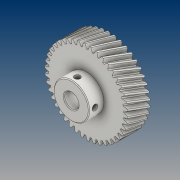
# Autodesk Inventor part: Final_Rang_Lon
Saved by Autodesk Inventor 2021 (Build 250183000, 183)
## iProperties
CustomPartVersion: 1
Created: 2024-04-07
Part Number: Final_Rang_Lon
Material: Steel
Document SubType Name: Modeling
Designer: Admin
Categories: <?xml version="1.0" encoding="UTF-16"?> <MemberInstance><Categories><FamilyTemplate><FamilyTemplateParameter ValueType="xs:double" Id="1" ObjectReferenceKey="da_z" ObjectType="kUserParameterObject"/><FamilyTemplateParameter ValueType="xs:double" Id="2" ObjectReferenceKey="da_b" ObjectType="kUserParameterObject"/><FamilyTemplateParameter ValueType="xs:double" Id="3" ObjectReferenceKey="da_beta" ObjectType="kUserParameterObject"/><FamilyTemplateParameter ValueType="xs:double" Id="4" ObjectReferenceKey="da_da" ObjectType="kUserParameterObject"/><FamilyTemplateParameter ValueType="xs:double" Id="5" ObjectReferenceKey="da_aw" ObjectType="kUserParameterObject"/><FamilyTemplateParameter ValueType="xs:string" Id="6" ObjectReferenceKey="EAIAABAAAACIAQAAAAAAAIAAAAAAAAAA" ObjectType="83910656" SubObjectId="SurfaceGeometry"/></FamilyTemplate><ParamToTemplateMap><ParamToTemplate CategoryParameter="//CategoryParameter[@InternalName='046C89C9-8512-4d59-83FE-43B91F4F132A']" TemplateParameter="1"/><ParamToTemplate CategoryParameter="//CategoryParameter[@InternalName='2552DF32-E462-4b46-AEBF-C6C7768E72AC']" TemplateParameter="2"/><ParamToTemplate CategoryParameter="//CategoryParameter[@InternalName='C9EE641D-15FC-4fae-A226-E94C4372FDD7']" TemplateParameter="3"/><ParamToTemplate><ParamToTemplate CategoryParameter="//CategoryParameter[@InternalName='00B6519A-459B-49c7-AD84-2E56D39A5744']" ConstantValue="-1.106123"/></ParamToTemplate><ParamToTemplate><ParamToTemplate CategoryParameter="//CategoryParameter[@InternalName='04B31F0E-C7A6-4894-AA32-9629BEFACF47']" ConstantValue="1.000000"/></ParamToTemplate><ParamToTemplate><ParamToTemplate CategoryParameter="//CategoryParameter[@InternalName='43CBEC2E-7847-49e7-A936-2F7889FCB2D9']" ConstantValue="0.250000"/></ParamToTemplate><ParamToTemplate><ParamToTemplate CategoryParameter="//CategoryParameter[@InternalName='B1EFC894-105D-4ebd-86BF-FA20ED196853']" ConstantValue="0.350000"/></ParamToTemplate><ParamToTemplate><ParamToTemplate CategoryParameter="//CategoryParameter[@InternalName='51175063-3D10-4879-93E8-6246FE8B403D']" ConstantValue="2060000000.000000"/></ParamToTemplate><ParamToTemplate><ParamToTemplate CategoryParameter="//CategoryParameter[@InternalName='A3A52E27-4454-46a9-B0BD-C932399B70AF']" ConstantValue="0.300000"/></ParamToTemplate><ParamToTemplate><ParamToTemplate CategoryParameter="//CategoryParameter[@InternalName='91B76062-C214-41d9-B1B9-14D2AB99603D']" ConstantValue="0.125000"/></ParamToTemplate><ParamToTemplate><ParamToTemplate CategoryParameter="//CategoryParameter[@InternalName='374E806E-8B8A-4dda-A9AA-1039D6500AD2']" ConstantValue="8.000000"/></ParamToTemplate><ParamToTemplate><ParamToTemplate CategoryParameter="//CategoryParameter[@InternalName='2D373A89-B862-43d6-8D0B-0CBF12AB9F6C']" ConstantValue="0.366519"/></ParamToTemplate><ParamToTemplate CategoryParameter="//CategoryParameter[@InternalName='37777632-D6A2-4fac-9D53-DB8ACD95C989']" TemplateParameter="4"/><ParamToTemplate CategoryParameter="//CategoryParameter[@InternalName='FD1017F1-B727-4f7e-9707-0F86F1FF9423']" TemplateParameter="5"/><ParamToTemplate><ParamToTemplate CategoryParameter="//CategoryParameter[@InternalName='9E1B4470-B2D3-4ff1-B813-535BB4CDF51A']" ConstantValue="3520000.000000"/></ParamToTemplate><ParamToTemplate><ParamToTemplate CategoryParameter="//CategoryParameter[@InternalName='F8452263-BFF6-458c-9FB1-07C4B99E95CD']" ConstantValue="11400000.000000"/></ParamToTemplate><ParamToTemplate><ParamToTemplate CategoryParameter="//CategoryParameter[@InternalName='3E3BB259-FD49-497f-8171-6EBC954A3479']" ConstantValue="2.000000"/></ParamToTemplate><ParamToTemplate CategoryParameter="//CategoryParameter[@InternalName='27C3BAF2-7550-4e4b-AE2C-0DB134B7D9B7']" TemplateParameter="6"/></ParamToTemplateMap><Category DisplayName="Gear" InternalName="DC85795E-93AB-48d5-8EEE-5A27447B64BD" Mnemonic="Gear"><CategoryParameter DisplayName="z" InternalName="046C89C9-8512-4d59-83FE-43B91F4F132A" Mnemonic="z"/><CategoryParameter DisplayName="b" InternalName="2552DF32-E462-4b46-AEBF-C6C7768E72AC" Mnemonic="b"/><CategoryParameter DisplayName="||b|" InternalName="C9EE641D-15FC-4fae-A226-E94C4372FDD7" Mnemonic="beta"/><CategoryParameter DisplayName="x" InternalName="00B6519A-459B-49c7-AD84-2E56D39A5744" Mnemonic="x"/><CategoryParameter DisplayName="a*" InternalName="04B31F0E-C7A6-4894-AA32-9629BEFACF47" Mnemonic="a"/><CategoryParameter DisplayName="c*" InternalName="43CBEC2E-7847-49e7-A936-2F7889FCB2D9" Mnemonic="c"/><CategoryParameter DisplayName="r|.f|*" InternalName="B1EFC894-105D-4ebd-86BF-FA20ED196853" Mnemonic="rf"/><CategoryParameter DisplayName="E" InternalName="51175063-3D10-4879-93E8-6246FE8B403D" Mnemonic="E"/><CategoryParameter DisplayName="||m|" InternalName="A3A52E27-4454-46a9-B0BD-C932399B70AF" Mnemonic="mi"/><Category DisplayName="SpurGear" InternalName="26C5A22E-A91E-4dfd-A3B3-23CCAFAE1764" Mnemonic="SpurGear"><CategoryParameter DisplayName="m" InternalName="91B76062-C214-41d9-B1B9-14D2AB99603D" Mnemonic="m"/><CategoryParameter DisplayName="P" InternalName="374E806E-8B8A-4dda-A9AA-1039D6500AD2" Mnemonic="PP"/><CategoryParameter DisplayName="||a|" InternalName="2D373A89-B862-43d6-8D0B-0CBF12AB9F6C" Mnemonic="alpha"/><CategoryParameter DisplayName="d|.a|" InternalName="37777632-D6A2-4fac-9D53-DB8ACD95C989" Mnemonic="da"/><CategoryParameter DisplayName="a|.w|" InternalName="FD1017F1-B727-4f7e-9707-0F86F1FF9423" Mnemonic="aw"/><CategoryParameter DisplayName="||s||.Flim|" InternalName="9E1B4470-B2D3-4ff1-B813-535BB4CDF51A" Mnemonic="sFlim"/><CategoryParameter DisplayName="||s||.Hlim|" InternalName="F8452263-BFF6-458c-9FB1-07C4B99E95CD" Mnemonic="sHlim"/><CategoryParameter DisplayName="type" InternalName="3E3BB259-FD49-497f-8171-6EBC954A3479" Mnemonic="type"/><CategoryParameter DisplayName="PitchDiameter" InternalName="27C3BAF2-7550-4e4b-AE2C-0DB134B7D9B7" Mnemonic="IDS_PITCHDIAM"/></Category></Category></Categories></MemberInstance>
Density: 1 g/cm^3
Appearance: Steel
Author: Admin
Autodesk Inventor part; units mm, degrees
ref_plane "YZ Plane" through (0, 0, 0) normal (1, 0, 0) x (0, 1, 0)
ref_plane "XZ Plane" through (0, 0, 0) normal (0, 1, 0) x (-1, 0, 0)
ref_plane "XY Plane" through (0, 0, 0) normal (0, 0, 1) x (1, 0, 0)
sketch "Sketch1" plane through (0, 0, 0) normal (0, 0, 1) x (1, 0, 0)
  circle A0 centre (0, 0) radius 27.6269
  dimension "d0" = 55.2538
  constraints: 1 centre point
  measures "d0" diameter of A0
extrude "Extrusion1" add sketch "Sketch1" along normal blind 15
ref_plane "Work Plane2" through (0, 0, 7.5) normal (0, 0, 1) x (1, 0, 0)
sketch "Sketch2" plane through (0, 0, 0) normal (0, 0, -1) x (-1, 0, 0)
  circle A0 centre (0, 0) radius 27.6269 projected
  circle A1 centre (0, 0) radius 27.9347
  dimension "d3" = 55.8693
  constraints: 1 centre point, 1 coincident
  measures "d3" diameter of A1
feature "Pitch Diameter" [suppressed]
ref_plane "Work Plane8" through (0, 0, 0) normal (0.9972038, 0.0747301, 0) x (0, 0, 1)
ref_plane "Work Plane9" through (0, 0, 0) normal (1, 0, 0) x (0, 1, 0)
spur gear teeth "Spur Gear" teeth 42 pitch diameter 55.8693 tip diameter 55.2538 root diameter 49.979 face width 15 helix angle 20 hand right start plane through (0, 0, 0) normal (0, 0, -1) x (-1, 0, 0)
sketch "Sketch3" plane through (0, 0, 15) normal (0, 0, 1) x (1, 0, 0)
  arc A0 (-12.6579, 24.5565) -> (-13.5673, 24.066) centre (0, 0) ccw projected
  arc A1 (-16.1765, 22.3957) -> (-17.0026, 21.7752) centre (0, 0) ccw projected
  arc A2 (-19.3337, 19.7345) -> (-20.0581, 18.9978) centre (0, 0) ccw projected
  arc A3 (-22.0591, 16.6326) -> (-22.6655, 15.7961) centre (0, 0) ccw projected
  arc A4 (-24.2916, 13.1591) -> (-24.7667, 12.2416) centre (0, 0) ccw projected
  arc A5 (-25.9816, 9.3916) -> (-26.3146, 8.4136) centre (0, 0) ccw projected
  arc A6 (-27.0911, 5.4144) -> (-27.2746, 4.3976) centre (0, 0) ccw projected
  arc A7 (-27.5955, 1.3162) -> (-27.6254, 0.2834) centre (0, 0) ccw projected
  arc A8 (-27.4835, -2.8114) -> (-27.3591, -3.8371) centre (0, 0) ccw projected
  arc A9 (-26.7575, -6.8762) -> (-26.4817, -7.8719) centre (0, 0) ccw projected
  arc A10 (-25.4338, -10.7874) -> (-25.0126, -11.7309) centre (0, 0) ccw projected
  arc A11 (-23.5419, -14.4576) -> (-22.9849, -15.3278) centre (0, 0) ccw projected
  arc A12 (-21.1242, -17.8049) -> (-20.4437, -18.5823) centre (0, 0) ccw projected
  arc A13 (-18.2346, -20.7544) -> (-17.4458, -21.4217) centre (0, 0) ccw projected
  arc A14 (-14.9376, -23.2403) -> (-14.0582, -23.7826) centre (0, 0) ccw projected
  arc A15 (-11.307, -25.2071) -> (-10.3565, -25.6122) centre (0, 0) ccw projected
  arc A16 (-7.4238, -26.6108) -> (-6.4236, -26.8697) centre (0, 0) ccw projected
  arc A17 (-3.3747, -27.42) -> (-2.3471, -27.527) centre (0, 0) ccw projected
  arc A18 (0.7497, -27.6167) -> (1.7818, -27.5694) centre (0, 0) ccw projected
  arc A19 (4.8574, -27.1965) -> (5.8709, -26.9959) centre (0, 0) ccw projected
  arc A20 (8.8566, -26.1688) -> (9.8289, -25.8193) centre (0, 0) ccw projected
  arc A21 (12.6579, -24.5565) -> (13.5673, -24.066) centre (0, 0) ccw projected
  arc A22 (16.1765, -22.3957) -> (17.0026, -21.7752) centre (0, 0) ccw projected
  arc A23 (19.3337, -19.7345) -> (20.0581, -18.9978) centre (0, 0) ccw projected
  arc A24 (22.0591, -16.6326) -> (22.6655, -15.7961) centre (0, 0) ccw projected
  arc A25 (24.2916, -13.1591) -> (24.7667, -12.2416) centre (0, 0) ccw projected
  arc A26 (25.9816, -9.3916) -> (26.3146, -8.4136) centre (0, 0) ccw projected
  arc A27 (27.0911, -5.4144) -> (27.2746, -4.3976) centre (0, 0) ccw projected
  arc A28 (27.5955, -1.3162) -> (27.6254, -0.2834) centre (0, 0) ccw projected
  arc A29 (27.4835, 2.8114) -> (27.3591, 3.8371) centre (0, 0) ccw projected
  arc A30 (26.7575, 6.8762) -> (26.4817, 7.8719) centre (0, 0) ccw projected
  arc A31 (25.4338, 10.7874) -> (25.0126, 11.7309) centre (0, 0) ccw projected
  arc A32 (23.5419, 14.4576) -> (22.9849, 15.3278) centre (0, 0) ccw projected
  arc A33 (21.1242, 17.8049) -> (20.4437, 18.5823) centre (0, 0) ccw projected
  arc A34 (18.2346, 20.7544) -> (17.4458, 21.4217) centre (0, 0) ccw projected
  arc A35 (14.9376, 23.2403) -> (14.0582, 23.7826) centre (0, 0) ccw projected
  arc A36 (11.307, 25.2071) -> (10.3565, 25.6122) centre (0, 0) ccw projected
  arc A37 (7.4238, 26.6108) -> (6.4236, 26.8697) centre (0, 0) ccw projected
  arc A38 (3.3747, 27.42) -> (2.3471, 27.527) centre (0, 0) ccw projected
  arc A39 (-0.7497, 27.6167) -> (-1.7818, 27.5694) centre (0, 0) ccw projected
  arc A40 (-4.8574, 27.1965) -> (-5.8709, 26.9959) centre (0, 0) ccw projected
  arc A41 (-8.8566, 26.1688) -> (-9.8289, 25.8193) centre (0, 0) ccw projected
  circle A42 centre (0, 0) radius 4.8
  circle A43 centre (0, 0) radius 11.8
  dimension "d49" = 7
  dimension "d50" = 9.6
  constraints: 2 centre point, 2 coincident, 126 other
  measures "d49" radial gap between concentric circles of A42 A43
  measures "d50" diameter of A42
extrude "Extrusion2" cut sketch "Sketch3" against normal through all contours A42
extrude "Extrusion3" add sketch "Sketch3" along normal blind 10
sketch "Sketch4" plane through (0, 0, 0) normal (1, 0, 0) x (0, 1, 0)
  line L0 (11.8, 25) -> (-11.8, 25) projected
  line L1 (-11.8, 15) -> (11.8, 15) projected
  line L2 (0, 15) -> (0, 25) construction
  circle A0 centre (0, 21) radius 1.9
  point P0 (0, 0)
  dimension "d55" = 4
  dimension "d56" = 3.8
  constraints: 2 end point, 2 midpoint, 1 centre point, 1 point on line
  measures "d55" distance from line of L0 A0.centre
  measures "d56" diameter of A0
extrude "Extrusion4" cut sketch "Sketch4" along normal through all
pattern_circular "Circular Pattern1" count 2 over 90 about axis through (0, 0, 15) along (0, 0, 1) of "Extrusion4"
chamfer "Chamfer1" distance 0.5 angle 45 1 edges at (-11.8, 0, 25)
chamfer "Chamfer2" distance 0.5 angle 45 2 edges at (-4.8, 0, 25) (-4.8, 0, 0)
equation "\"d0\" = da_da"
equation "\"d1\" = da_b"
equation "\"d3\" = da_d"
equation "\"d16\" = da_aw"
equation "\"d43\" = da_aw"
equation "\"d46\" = da_aw"
equation "\"da_da\" = 55.253778"
equation "\"da_b\" = 15"
equation "\"da_d\" = 55.869333"
equation "\"da_aw\" = 45"
body "Solid1"
body "Srf1"
